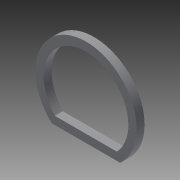
# Autodesk Inventor part: TSOP Ring
Saved by Autodesk Inventor 2015 (Build 190159000, 159)
## iProperties
Created: 2016-08-09
Part Number: TSOP Ring
Material: Generic
Document SubType Name: Modeling
Designer: James Yelland
Density: 1 g/cm^3
Appearance: Default
Author: James Yelland
Autodesk Inventor part; units mm, degrees
ref_plane "YZ Plane" through (0, 0, 0) normal (1, 0, 0) x (0, 1, 0)
ref_plane "XZ Plane" through (0, 0, 0) normal (0, 1, 0) x (-1, 0, 0)
ref_plane "XY Plane" through (0, 0, 0) normal (0, 0, 1) x (1, 0, 0)
sketch "Sketch1" plane through (0, 0, 0) normal (0, 1, 0) x (-1, 0, 0)
  line L0 (0, -70) -> (-64.2262, -70)
  line L1 (0, -70) -> (64.2262, -70)
  line L2 (0, -55) -> (58.0948, -55)
  line L3 (0, -55) -> (-58.0948, -55)
  arc A0 (64.2262, -70) -> (-64.2262, -70) centre (0, 0) ccw
  arc A1 (58.0948, -55) -> (-58.0948, -55) centre (0, -0.7993) ccw
  constraints: 8 end point, 4 point on circle, 2 centre point, 2 point on line, 1 coincident
extrude "Extrusion1" add sketch "Sketch1" along normal blind 15
fillet "Fillet1" radius 2 4 edges at (64.2262, 7.5, -70) (-64.2262, 7.5, -70) (58.0948, 7.5, -55) (-58.0948, 7.5, -55)
sketch "Sketch2" plane through (0, 15, 0) normal (0, 1, 0) x (1, 0, 0)
  line L0 (-5.4, 64.95) -> (-5.4, 60.15)
  line L1 (-5.4, 60.15) -> (5.4, 60.15)
  line L2 (5.4, 60.15) -> (5.4, 64.95)
  arc A0 (2.5807, 64.95) -> (-2.5807, 64.95) centre (0, 64) ccw
  line L3 (-5.4, 64.95) -> (-2.5807, 64.95)
  line L4 (2.5807, 64.95) -> (5.4, 64.95)
  line L5 (0, 66.75) -> (0, 64)
  line L6 (0, 64) -> (0, 70)
  line L7 (-26.3195, 63.5285) -> (-24.8363, 58.9634)
  line L8 (-20.8903, 64.2937) -> (-22.7444, 70)
  line L9 (-21.7401, 66.9091) -> (-20.8903, 64.2937)
  arc A1 (-18.7295, 65.9946) -> (-23.6382, 64.3997) centre (-20.8903, 64.2937) ccw
  line L10 (-18.7295, 65.9946) -> (-16.0481, 66.8659)
  line L11 (-24.8363, 58.9634) -> (-14.5649, 62.3008)
  line L12 (-14.5649, 62.3008) -> (-16.0481, 66.8659)
  line L13 (-26.3195, 63.5285) -> (-23.6382, 64.3997)
  line L14 (-52.2584, 62.7404) -> (-49.437, 58.8571)
  line L15 (-47.3313, 65.1459) -> (-50.858, 70)
  line L16 (-48.9477, 67.3707) -> (-47.3313, 65.1459)
  arc A2 (-45.8018, 67.4314) -> (-49.9775, 64.3976) centre (-47.3313, 65.1459) ccw
  line L17 (-45.8018, 67.4314) -> (-43.521, 69.0885)
  line L18 (-49.437, 58.8571) -> (-40.6996, 65.2052)
  line L19 (-40.6996, 65.2052) -> (-43.521, 69.0885)
  line L20 (-52.2584, 62.7404) -> (-49.9775, 64.3976)
  line L21 (-75.9451, 48.5026) -> (-72.0618, 45.6812)
  line L22 (-72.0025, 52.3129) -> (-76.8566, 55.8396)
  line L23 (-74.2273, 53.9293) -> (-72.0025, 52.3129)
  arc A3 (-71.2542, 54.9591) -> (-74.288, 50.7835) centre (-72.0025, 52.3129) ccw
  line L24 (-71.2542, 54.9591) -> (-69.597, 57.24)
  line L25 (-72.0618, 45.6812) -> (-65.7138, 54.4186)
  line L26 (-65.7138, 54.4186) -> (-69.597, 57.24)
  line L27 (-75.9451, 48.5026) -> (-74.288, 50.7835)
  line L28 (-87.2162, 22.6604) -> (-82.6512, 21.1771)
  line L29 (-84.644, 27.5025) -> (-90.3504, 29.3566)
  line L30 (-87.2594, 28.3523) -> (-84.644, 27.5025)
  arc A4 (-84.7501, 30.2505) -> (-86.345, 25.3417) centre (-84.644, 27.5025) ccw
  line L31 (-84.7501, 30.2505) -> (-83.8788, 32.9318)
  line L32 (-82.6512, 21.1771) -> (-79.3138, 31.4485)
  line L33 (-79.3138, 31.4485) -> (-83.8788, 32.9318)
  line L34 (-87.2162, 22.6604) -> (-86.345, 25.3417)
  line L35 (-89.95, -5.4) -> (-85.15, -5.4)
  line L36 (-89, 0) -> (-95, 0)
  line L37 (-91.75, 0) -> (-89, 0)
  arc A5 (-89.95, 2.5807) -> (-89.95, -2.5807) centre (-89, 0) ccw
  line L38 (-89.95, 2.5807) -> (-89.95, 5.4)
  line L39 (-85.15, -5.4) -> (-85.15, 5.4)
  line L40 (-85.15, 5.4) -> (-89.95, 5.4)
  line L41 (-89.95, -5.4) -> (-89.95, -2.5807)
  line L42 (-83.8788, -32.9318) -> (-79.3138, -31.4485)
  line L43 (-84.644, -27.5025) -> (-90.3504, -29.3566)
  line L44 (-87.2594, -28.3523) -> (-84.644, -27.5025)
  arc A6 (-86.345, -25.3417) -> (-84.7501, -30.2505) centre (-84.644, -27.5025) ccw
  line L45 (-86.345, -25.3417) -> (-87.2162, -22.6604)
  line L46 (-79.3138, -31.4485) -> (-82.6512, -21.1771)
  line L47 (-82.6512, -21.1771) -> (-87.2162, -22.6604)
  line L48 (-83.8788, -32.9318) -> (-84.7501, -30.2505)
  line L49 (-69.597, -57.24) -> (-65.7138, -54.4186)
  line L50 (-72.0025, -52.3129) -> (-76.8566, -55.8396)
  line L51 (-74.2273, -53.9293) -> (-72.0025, -52.3129)
  arc A7 (-74.288, -50.7835) -> (-71.2542, -54.9591) centre (-72.0025, -52.3129) ccw
  line L52 (-74.288, -50.7835) -> (-75.9451, -48.5026)
  line L53 (-65.7138, -54.4186) -> (-72.0618, -45.6812)
  line L54 (-72.0618, -45.6812) -> (-75.9451, -48.5026)
  line L55 (-69.597, -57.24) -> (-71.2542, -54.9591)
  line L56 (-48.5026, -75.9451) -> (-45.6812, -72.0618)
  line L57 (-52.3129, -72.0025) -> (-55.8396, -76.8566)
  line L58 (-53.9293, -74.2273) -> (-52.3129, -72.0025)
  arc A8 (-54.9591, -71.2542) -> (-50.7835, -74.288) centre (-52.3129, -72.0025) ccw
  line L59 (-54.9591, -71.2542) -> (-57.24, -69.597)
  line L60 (-45.6812, -72.0618) -> (-54.4186, -65.7138)
  line L61 (-54.4186, -65.7138) -> (-57.24, -69.597)
  line L62 (-48.5026, -75.9451) -> (-50.7835, -74.288)
  line L63 (-22.6604, -87.2162) -> (-21.1771, -82.6512)
  line L64 (-27.5025, -84.644) -> (-29.3566, -90.3504)
  line L65 (-28.3523, -87.2594) -> (-27.5025, -84.644)
  arc A9 (-30.2505, -84.7501) -> (-25.3417, -86.345) centre (-27.5025, -84.644) ccw
  line L66 (-30.2505, -84.7501) -> (-32.9318, -83.8788)
  line L67 (-21.1771, -82.6512) -> (-31.4485, -79.3138)
  line L68 (-31.4485, -79.3138) -> (-32.9318, -83.8788)
  line L69 (-22.6604, -87.2162) -> (-25.3417, -86.345)
  line L70 (5.4, -89.95) -> (5.4, -85.15)
  line L71 (0, -89) -> (0, -95)
  line L72 (0, -91.75) -> (0, -89)
  arc A10 (-2.5807, -89.95) -> (2.5807, -89.95) centre (0, -89) ccw
  line L73 (-2.5807, -89.95) -> (-5.4, -89.95)
  line L74 (5.4, -85.15) -> (-5.4, -85.15)
  line L75 (-5.4, -85.15) -> (-5.4, -89.95)
  line L76 (5.4, -89.95) -> (2.5807, -89.95)
  line L77 (32.9318, -83.8788) -> (31.4485, -79.3138)
  line L78 (27.5025, -84.644) -> (29.3566, -90.3504)
  line L79 (28.3523, -87.2594) -> (27.5025, -84.644)
  arc A11 (25.3417, -86.345) -> (30.2505, -84.7501) centre (27.5025, -84.644) ccw
  line L80 (25.3417, -86.345) -> (22.6604, -87.2162)
  line L81 (31.4485, -79.3138) -> (21.1771, -82.6512)
  line L82 (21.1771, -82.6512) -> (22.6604, -87.2162)
  line L83 (32.9318, -83.8788) -> (30.2505, -84.7501)
  line L84 (57.24, -69.597) -> (54.4186, -65.7138)
  line L85 (52.3129, -72.0025) -> (55.8396, -76.8566)
  line L86 (53.9293, -74.2273) -> (52.3129, -72.0025)
  arc A12 (50.7835, -74.288) -> (54.9591, -71.2542) centre (52.3129, -72.0025) ccw
  line L87 (50.7835, -74.288) -> (48.5026, -75.9451)
  line L88 (54.4186, -65.7138) -> (45.6812, -72.0618)
  line L89 (45.6812, -72.0618) -> (48.5026, -75.9451)
  line L90 (57.24, -69.597) -> (54.9591, -71.2542)
  line L91 (75.9451, -48.5026) -> (72.0618, -45.6812)
  line L92 (72.0025, -52.3129) -> (76.8566, -55.8396)
  line L93 (74.2273, -53.9293) -> (72.0025, -52.3129)
  arc A13 (71.2542, -54.9591) -> (74.288, -50.7835) centre (72.0025, -52.3129) ccw
  line L94 (71.2542, -54.9591) -> (69.597, -57.24)
  line L95 (72.0618, -45.6812) -> (65.7138, -54.4186)
  line L96 (65.7138, -54.4186) -> (69.597, -57.24)
  line L97 (75.9451, -48.5026) -> (74.288, -50.7835)
  line L98 (87.2162, -22.6604) -> (82.6512, -21.1771)
  line L99 (84.644, -27.5025) -> (90.3504, -29.3566)
  line L100 (87.2594, -28.3523) -> (84.644, -27.5025)
  arc A14 (84.7501, -30.2505) -> (86.345, -25.3417) centre (84.644, -27.5025) ccw
  line L101 (84.7501, -30.2505) -> (83.8788, -32.9318)
  line L102 (82.6512, -21.1771) -> (79.3138, -31.4485)
  line L103 (79.3138, -31.4485) -> (83.8788, -32.9318)
  line L104 (87.2162, -22.6604) -> (86.345, -25.3417)
  line L105 (89.95, 5.4) -> (85.15, 5.4)
  line L106 (89, 0) -> (95, 0)
  line L107 (91.75, 0) -> (89, 0)
  arc A15 (89.95, -2.5807) -> (89.95, 2.5807) centre (89, 0) ccw
  line L108 (89.95, -2.5807) -> (89.95, -5.4)
  line L109 (85.15, 5.4) -> (85.15, -5.4)
  line L110 (85.15, -5.4) -> (89.95, -5.4)
  line L111 (89.95, 5.4) -> (89.95, 2.5807)
  line L112 (83.8788, 32.9318) -> (79.3138, 31.4485)
  line L113 (84.644, 27.5025) -> (90.3504, 29.3566)
  line L114 (87.2594, 28.3523) -> (84.644, 27.5025)
  arc A16 (86.345, 25.3417) -> (84.7501, 30.2505) centre (84.644, 27.5025) ccw
  line L115 (86.345, 25.3417) -> (87.2162, 22.6604)
  line L116 (79.3138, 31.4485) -> (82.6512, 21.1771)
  line L117 (82.6512, 21.1771) -> (87.2162, 22.6604)
  line L118 (83.8788, 32.9318) -> (84.7501, 30.2505)
  line L119 (69.597, 57.24) -> (65.7138, 54.4186)
  line L120 (72.0025, 52.3129) -> (76.8566, 55.8396)
  line L121 (74.2273, 53.9293) -> (72.0025, 52.3129)
  arc A17 (74.288, 50.7835) -> (71.2542, 54.9591) centre (72.0025, 52.3129) ccw
  line L122 (74.288, 50.7835) -> (75.9451, 48.5026)
  line L123 (65.7138, 54.4186) -> (72.0618, 45.6812)
  line L124 (72.0618, 45.6812) -> (75.9451, 48.5026)
  line L125 (69.597, 57.24) -> (71.2542, 54.9591)
  line L126 (43.521, 69.0885) -> (40.6996, 65.2052)
  line L127 (47.3313, 65.1459) -> (50.858, 70)
  line L128 (48.9477, 67.3707) -> (47.3313, 65.1459)
  arc A18 (49.9775, 64.3976) -> (45.8018, 67.4314) centre (47.3313, 65.1459) ccw
  line L129 (49.9775, 64.3976) -> (52.2584, 62.7404)
  line L130 (40.6996, 65.2052) -> (49.437, 58.8571)
  line L131 (49.437, 58.8571) -> (52.2584, 62.7404)
  line L132 (43.521, 69.0885) -> (45.8018, 67.4314)
  line L133 (16.0481, 66.8659) -> (14.5649, 62.3008)
  line L134 (20.8903, 64.2937) -> (22.7444, 70)
  line L135 (21.7401, 66.9091) -> (20.8903, 64.2937)
  arc A19 (23.6382, 64.3997) -> (18.7295, 65.9946) centre (20.8903, 64.2937) ccw
  line L136 (23.6382, 64.3997) -> (26.3195, 63.5285)
  line L137 (14.5649, 62.3008) -> (24.8363, 58.9634)
  line L138 (24.8363, 58.9634) -> (26.3195, 63.5285)
  line L139 (16.0481, 66.8659) -> (18.7295, 65.9946)
  line L140 (63.4429, 70) -> (-63.4429, 70)
  line L141 (63.4429, 70) -> (-63.4429, 70) projected
  point P0 (0, 0)
  dimension "d20" = 360
  constraints: 282 end point, 41 point on circle, 20 centre point, 1 other
extrude "Extrusion2" cut sketch "Sketch2" against normal blind 13
body "Solid1"
